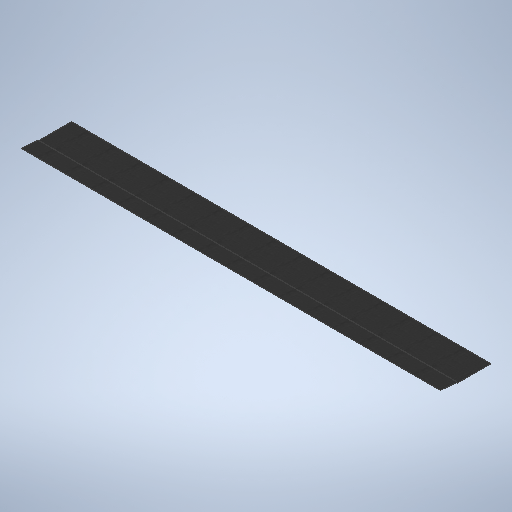
# Autodesk Inventor part: Underlayment_Over_Intake_Vent
Saved by Autodesk Inventor 2025.1 (Build 291241020, 241B)
## iProperties
Created: 2024-10-02
Part Number: Underlayment_Over_Intake_Vent
Material: Generic
Document SubType Name: Modeling
Designer: Tom
Density: 1 g/cm^3
Appearance: Asphalt 2
Author: Tom
Autodesk Inventor part; units mm, degrees
ref_plane "YZ Plane" through (0, 0, 0) normal (1, 0, 0) x (0, 1, 0)
ref_plane "XZ Plane" through (0, 0, 0) normal (0, 1, 0) x (-1, 0, 0)
ref_plane "XY Plane" through (0, 0, 0) normal (0, 0, 1) x (1, 0, 0)
sketch "Sketch1" plane through (0, 0, 0) normal (1, 0, 0) x (0, 1, 0)
  line L0 (0, 0) -> (0, 597.7382)
  line L1 (0, 0) -> (3.175, 0)
  line L2 (3.175, 0) -> (3.175, 594.5632)
  line L3 (3.175, 594.5632) -> (9.906, 594.5632)
  line L4 (9.906, 594.5632) -> (15.756, 595.9828)
  line L5 (0, 597.7382) -> (9.5263, 597.7382)
  line L6 (9.5263, 597.7382) -> (12.7824, 598.5283)
  line L7 (41.2921, 902.0052) -> (15.756, 595.9828)
  line L8 (12.7824, 598.5283) -> (38.1281, 902.2692)
  line L9 (38.1281, 902.2692) -> (41.2921, 902.0052)
  dimension "d0" = 594.5632
  dimension "d1" = 3.175
  dimension "d2" = 6.731
  dimension "d7" = 3.175
  dimension "d8" = 6.0198
  dimension "d9" = 166.36
  dimension "d10" = 3.175
  dimension "d11" = 108.41
  dimension "d12" = 3.175
  dimension "d13" = 307.086
  constraints: 20 end point, 4 perpendicular, 2 parallel, 1 horizontal, 1 vertical
  measures "d0" distance of L1.end L2.end
  measures "d1" distance between parallel lines of L2 L0
  measures "d2" distance of L2.end L3.end
  measures "d7" distance between parallel lines of L5 L3
  measures "d8" distance of L3.end L4.end
  measures "d9" angle of L3 L4
  measures "d10" distance between parallel lines of L6 L4
  measures "d11" angle of L4 L7
  measures "d12" distance between parallel lines of L7 L8
  measures "d13" distance of L7.start L4.end
extrude "Extrusion1" add sketch "Sketch1" along normal blind 7494.905
body "Solid1"
